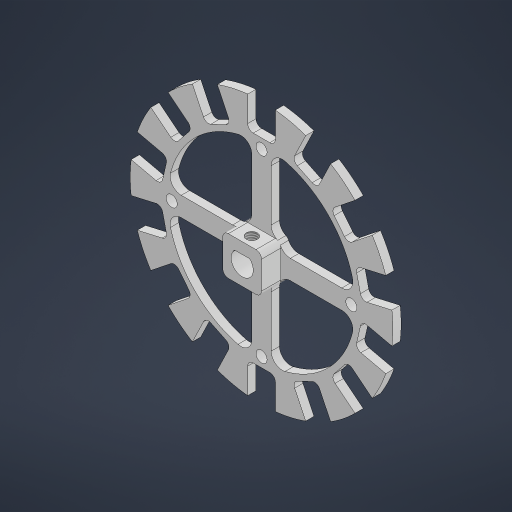
# Autodesk Inventor part: OmniFrame_A
Saved by Autodesk Inventor 2024.2 (Build 282272000, 272)
## iProperties
Created: 2023-12-20
Part Number: OmniFrame_A
Material: 一般
Document SubType Name: Modeling
Designer: Hanaoka
Density: 1 g/cm^3
Appearance: 既定
Author: Hanaoka
Autodesk Inventor part; units mm, degrees
ref_plane "YZ Plane" through (0, 0, 0) normal (1, 0, 0) x (0, 1, 0)
ref_plane "XZ Plane" through (0, 0, 0) normal (0, 1, 0) x (-1, 0, 0)
ref_plane "XY Plane" through (0, 0, 0) normal (0, 0, 1) x (1, 0, 0)
derived "OmniFrame_B.ipt"
sketch "スケッチ1" plane through (0, 0, 0) normal (0, 0, 1) x (1, 0, 0)
  circle A0 centre (0, 0) radius 25 construction
  line L0 (-2.5, 24.874686) -> (-2.5, 19)
  line L1 (-1.5, 18) -> (1.5, 18)
  line L2 (2.5, 19) -> (2.5, 24.874686)
  line L3 (0, 25) -> (0, 18) construction
  line L4 (-2.5, 23.025) -> (-3, 23.025)
  line L5 (-4, 22.025) -> (-4, 21.975)
  line L6 (-3, 20.975) -> (-2.5, 20.975)
  line L7 (2.5, 23.025) -> (3, 23.025)
  line L8 (4, 22.025) -> (4, 21.975)
  line L9 (3, 20.975) -> (2.5, 20.975)
  arc A1 (-3, 23.025) -> (-4, 22.025) centre (-3, 22.025) ccw
  arc A2 (-4, 21.975) -> (-3, 20.975) centre (-3, 21.975) ccw
  arc A3 (4, 22.025) -> (3, 23.025) centre (3, 22.025) ccw
  arc A4 (3, 20.975) -> (4, 21.975) centre (3, 21.975) ccw
  arc A5 (-2.5, 19) -> (-1.5, 18) centre (-1.5, 19) ccw
  arc A6 (1.5, 18) -> (2.5, 19) centre (1.5, 19) ccw
  arc A7 (-10.496213, 16.033699) -> (-9.161361, 15.566614) centre (-9.595244, 16.467583) ccw
  arc A8 (-6.458454, 16.868265) -> (-5.991369, 18.203118) centre (-6.892338, 17.769234) ccw
  line L10 (-9.161361, 15.566614) -> (-6.458454, 16.868265)
  line L11 (-6.397805, 20.199473) -> (-6.848289, 19.982531)
  arc A9 (-6.397805, 20.199473) -> (-5.93072, 21.534326) centre (-6.831689, 21.100442) ccw
  line L12 (-5.952414, 21.579374) -> (-5.93072, 21.534326)
  arc A10 (-5.952414, 21.579374) -> (-7.287266, 22.046459) centre (-6.853383, 21.145491) ccw
  line L13 (-7.737751, 21.829518) -> (-7.287266, 22.046459)
  line L14 (-11.803618, 17.596171) -> (-11.353134, 17.813113)
  line L15 (-5.991369, 18.203118) -> (-8.5403, 23.496027)
  line L16 (-10.847093, 22.524222) -> (-7.809907, 16.21744) construction
  line L17 (-13.045144, 21.326608) -> (-10.496213, 16.033699)
  arc A11 (-13.138471, 18.063256) -> (-11.803618, 17.596171) centre (-12.237502, 18.49714) ccw
  line L18 (-12.242595, 19.660099) -> (-12.69308, 19.443157)
  line L19 (-13.160165, 18.108304) -> (-13.138471, 18.063256)
  arc A12 (-12.69308, 19.443157) -> (-13.160165, 18.108304) centre (-12.259196, 18.542188) ccw
  arc A13 (-16.413523, 9.891728) -> (-15.008201, 10.050069) centre (-15.790033, 10.673559) ccw
  arc A14 (-13.137732, 12.395564) -> (-13.296074, 13.800885) centre (-13.919563, 13.019053) ccw
  line L20 (-15.008201, 10.050069) -> (-13.137732, 12.395564)
  line L21 (-14.528446, 15.423193) -> (-14.840191, 15.032277)
  arc A15 (-14.528446, 15.423193) -> (-14.686788, 16.828514) centre (-15.310277, 16.046683) ccw
  line L22 (-14.725879, 16.859689) -> (-14.686788, 16.828514)
  arc A16 (-14.725879, 16.859689) -> (-16.1312, 16.701347) centre (-15.349369, 16.077857) ccw
  line L23 (-16.442945, 16.310431) -> (-16.1312, 16.701347)
  line L24 (-18.269385, 10.732204) -> (-17.95764, 11.12312)
  line L25 (-13.296074, 13.800885) -> (-17.889088, 17.463692)
  line L26 (-19.545787, 15.587245) -> (-14.072967, 11.222816) construction
  line L27 (-21.006537, 13.554534) -> (-16.413523, 9.891728)
  arc A17 (-19.674706, 10.573862) -> (-18.269385, 10.732204) centre (-19.051216, 11.355694) ccw
  line L28 (-19.560394, 12.401274) -> (-19.872139, 12.010358)
  line L29 (-19.713798, 10.605037) -> (-19.674706, 10.573862)
  arc A18 (-19.872139, 12.010358) -> (-19.713798, 10.605037) centre (-19.090308, 11.386868) ccw
  arc A19 (-19.079933, 1.790578) -> (-17.882484, 2.542985) centre (-18.857412, 2.765506) ccw
  arc A20 (-17.214921, 5.467769) -> (-17.967328, 6.665218) centre (-18.189849, 5.69029) ccw
  line L30 (-17.882484, 2.542985) -> (-17.214921, 5.467769)
  line L31 (-19.78155, 7.59216) -> (-19.892811, 7.104696)
  arc A21 (-19.78155, 7.59216) -> (-20.533957, 8.789609) centre (-20.756478, 7.814681) ccw
  line L32 (-20.582704, 8.800735) -> (-20.533957, 8.789609)
  arc A22 (-20.582704, 8.800735) -> (-21.780152, 8.048328) centre (-20.805224, 7.825807) ccw
  line L33 (-21.891413, 7.560864) -> (-21.780152, 8.048328)
  line L34 (-21.116676, 1.742593) -> (-21.005415, 2.230057)
  line L35 (-17.967328, 6.665218) -> (-23.694723, 7.972458)
  line L36 (-24.373198, 5.563023) -> (-17.548702, 4.005377) construction
  line L37 (-24.807328, 3.097819) -> (-19.079933, 1.790578)
  arc A23 (-22.314125, 0.990186) -> (-21.116676, 1.742593) centre (-22.091604, 1.965114) ccw
  line L38 (-23.004018, 2.686225) -> (-23.115278, 2.198761)
  line L39 (-22.362871, 1.001312) -> (-22.314125, 0.990186)
  arc A24 (-23.115278, 2.198761) -> (-22.362871, 1.001312) centre (-22.14035, 1.97624) ccw
  arc A25 (-17.967328, -6.665218) -> (-17.214921, -5.467769) centre (-18.189849, -5.69029) ccw
  arc A26 (-17.882484, -2.542985) -> (-19.079933, -1.790578) centre (-18.857412, -2.765506) ccw
  line L40 (-17.214921, -5.467769) -> (-17.882484, -2.542985)
  line L41 (-21.116676, -1.742593) -> (-21.005415, -2.230057)
  arc A27 (-21.116676, -1.742593) -> (-22.314125, -0.990186) centre (-22.091604, -1.965114) ccw
  line L42 (-22.362871, -1.001312) -> (-22.314125, -0.990186)
  arc A28 (-22.362871, -1.001312) -> (-23.115278, -2.198761) centre (-22.14035, -1.97624) ccw
  line L43 (-23.004018, -2.686225) -> (-23.115278, -2.198761)
  line L44 (-19.78155, -7.59216) -> (-19.892811, -7.104696)
  line L45 (-19.079933, -1.790578) -> (-24.807328, -3.097819)
  line L46 (-24.373198, -5.563023) -> (-17.548702, -4.005377) construction
  line L47 (-23.694723, -7.972458) -> (-17.967328, -6.665218)
  arc A29 (-20.533957, -8.789609) -> (-19.78155, -7.59216) centre (-20.756478, -7.814681) ccw
  line L48 (-21.891413, -7.560864) -> (-21.780152, -8.048328)
  line L49 (-20.582704, -8.800735) -> (-20.533957, -8.789609)
  arc A30 (-21.780152, -8.048328) -> (-20.582704, -8.800735) centre (-20.805224, -7.825807) ccw
  arc A31 (-13.296074, -13.800885) -> (-13.137732, -12.395564) centre (-13.919563, -13.019053) ccw
  arc A32 (-15.008201, -10.050069) -> (-16.413523, -9.891728) centre (-15.790033, -10.673559) ccw
  line L50 (-13.137732, -12.395564) -> (-15.008201, -10.050069)
  line L51 (-18.269385, -10.732204) -> (-17.95764, -11.12312)
  arc A33 (-18.269385, -10.732204) -> (-19.674706, -10.573862) centre (-19.051216, -11.355694) ccw
  line L52 (-19.713798, -10.605037) -> (-19.674706, -10.573862)
  arc A34 (-19.713798, -10.605037) -> (-19.872139, -12.010358) centre (-19.090308, -11.386868) ccw
  line L53 (-19.560394, -12.401274) -> (-19.872139, -12.010358)
  line L54 (-14.528446, -15.423193) -> (-14.840191, -15.032277)
  line L55 (-16.413523, -9.891728) -> (-21.006537, -13.554534)
  line L56 (-19.545787, -15.587245) -> (-14.072967, -11.222816) construction
  line L57 (-17.889088, -17.463692) -> (-13.296074, -13.800885)
  arc A35 (-14.686788, -16.828514) -> (-14.528446, -15.423193) centre (-15.310277, -16.046683) ccw
  line L58 (-16.442945, -16.310431) -> (-16.1312, -16.701347)
  line L59 (-14.725879, -16.859689) -> (-14.686788, -16.828514)
  arc A36 (-16.1312, -16.701347) -> (-14.725879, -16.859689) centre (-15.349369, -16.077857) ccw
  arc A37 (-5.991369, -18.203118) -> (-6.458454, -16.868265) centre (-6.892338, -17.769234) ccw
  arc A38 (-9.161361, -15.566614) -> (-10.496213, -16.033699) centre (-9.595244, -16.467583) ccw
  line L60 (-6.458454, -16.868265) -> (-9.161361, -15.566614)
  line L61 (-11.803618, -17.596171) -> (-11.353134, -17.813113)
  arc A39 (-11.803618, -17.596171) -> (-13.138471, -18.063256) centre (-12.237502, -18.49714) ccw
  line L62 (-13.160165, -18.108304) -> (-13.138471, -18.063256)
  arc A40 (-13.160165, -18.108304) -> (-12.69308, -19.443157) centre (-12.259196, -18.542188) ccw
  line L63 (-12.242595, -19.660099) -> (-12.69308, -19.443157)
  line L64 (-6.397805, -20.199473) -> (-6.848289, -19.982531)
  line L65 (-10.496213, -16.033699) -> (-13.045144, -21.326608)
  line L66 (-10.847093, -22.524222) -> (-7.809907, -16.21744) construction
  line L67 (-8.5403, -23.496027) -> (-5.991369, -18.203118)
  arc A41 (-5.93072, -21.534326) -> (-6.397805, -20.199473) centre (-6.831689, -21.100442) ccw
  line L68 (-7.737751, -21.829518) -> (-7.287266, -22.046459)
  line L69 (-5.952414, -21.579374) -> (-5.93072, -21.534326)
  arc A42 (-7.287266, -22.046459) -> (-5.952414, -21.579374) centre (-6.853383, -21.145491) ccw
  arc A43 (2.5, -19) -> (1.5, -18) centre (1.5, -19) ccw
  arc A44 (-1.5, -18) -> (-2.5, -19) centre (-1.5, -19) ccw
  line L70 (1.5, -18) -> (-1.5, -18)
  line L71 (-3, -20.975) -> (-2.5, -20.975)
  arc A45 (-3, -20.975) -> (-4, -21.975) centre (-3, -21.975) ccw
  line L72 (-4, -22.025) -> (-4, -21.975)
  arc A46 (-4, -22.025) -> (-3, -23.025) centre (-3, -22.025) ccw
  line L73 (-2.5, -23.025) -> (-3, -23.025)
  line L74 (3, -20.975) -> (2.5, -20.975)
  line L75 (-2.5, -19) -> (-2.5, -24.874686)
  line L76 (0, -25) -> (0, -18) construction
  line L77 (2.5, -24.874686) -> (2.5, -19)
  arc A47 (4, -21.975) -> (3, -20.975) centre (3, -21.975) ccw
  line L78 (2.5, -23.025) -> (3, -23.025)
  line L79 (4, -22.025) -> (4, -21.975)
  arc A48 (3, -23.025) -> (4, -22.025) centre (3, -22.025) ccw
  arc A49 (10.496213, -16.033699) -> (9.161361, -15.566614) centre (9.595244, -16.467583) ccw
  arc A50 (6.458454, -16.868265) -> (5.991369, -18.203118) centre (6.892338, -17.769234) ccw
  line L80 (9.161361, -15.566614) -> (6.458454, -16.868265)
  line L81 (6.397805, -20.199473) -> (6.848289, -19.982531)
  arc A51 (6.397805, -20.199473) -> (5.93072, -21.534326) centre (6.831689, -21.100442) ccw
  line L82 (5.952414, -21.579374) -> (5.93072, -21.534326)
  arc A52 (5.952414, -21.579374) -> (7.287266, -22.046459) centre (6.853383, -21.145491) ccw
  line L83 (7.737751, -21.829518) -> (7.287266, -22.046459)
  line L84 (11.803618, -17.596171) -> (11.353134, -17.813113)
  line L85 (5.991369, -18.203118) -> (8.5403, -23.496027)
  line L86 (10.847093, -22.524222) -> (7.809907, -16.21744) construction
  line L87 (13.045144, -21.326608) -> (10.496213, -16.033699)
  arc A53 (13.138471, -18.063256) -> (11.803618, -17.596171) centre (12.237502, -18.49714) ccw
  line L88 (12.242595, -19.660099) -> (12.69308, -19.443157)
  line L89 (13.160165, -18.108304) -> (13.138471, -18.063256)
  arc A54 (12.69308, -19.443157) -> (13.160165, -18.108304) centre (12.259196, -18.542188) ccw
  arc A55 (16.413523, -9.891728) -> (15.008201, -10.050069) centre (15.790033, -10.673559) ccw
  arc A56 (13.137732, -12.395564) -> (13.296074, -13.800885) centre (13.919563, -13.019053) ccw
  line L90 (15.008201, -10.050069) -> (13.137732, -12.395564)
  line L91 (14.528446, -15.423193) -> (14.840191, -15.032277)
  arc A57 (14.528446, -15.423193) -> (14.686788, -16.828514) centre (15.310277, -16.046683) ccw
  line L92 (14.725879, -16.859689) -> (14.686788, -16.828514)
  arc A58 (14.725879, -16.859689) -> (16.1312, -16.701347) centre (15.349369, -16.077857) ccw
  line L93 (16.442945, -16.310431) -> (16.1312, -16.701347)
  line L94 (18.269385, -10.732204) -> (17.95764, -11.12312)
  line L95 (13.296074, -13.800885) -> (17.889088, -17.463692)
  line L96 (19.545787, -15.587245) -> (14.072967, -11.222816) construction
  line L97 (21.006537, -13.554534) -> (16.413523, -9.891728)
  arc A59 (19.674706, -10.573862) -> (18.269385, -10.732204) centre (19.051216, -11.355694) ccw
  line L98 (19.560394, -12.401274) -> (19.872139, -12.010358)
  line L99 (19.713798, -10.605037) -> (19.674706, -10.573862)
  arc A60 (19.872139, -12.010358) -> (19.713798, -10.605037) centre (19.090308, -11.386868) ccw
  arc A61 (19.079933, -1.790578) -> (17.882484, -2.542985) centre (18.857412, -2.765506) ccw
  arc A62 (17.214921, -5.467769) -> (17.967328, -6.665218) centre (18.189849, -5.69029) ccw
  line L100 (17.882484, -2.542985) -> (17.214921, -5.467769)
  line L101 (19.78155, -7.59216) -> (19.892811, -7.104696)
  arc A63 (19.78155, -7.59216) -> (20.533957, -8.789609) centre (20.756478, -7.814681) ccw
  line L102 (20.582704, -8.800735) -> (20.533957, -8.789609)
  arc A64 (20.582704, -8.800735) -> (21.780152, -8.048328) centre (20.805224, -7.825807) ccw
  line L103 (21.891413, -7.560864) -> (21.780152, -8.048328)
  line L104 (21.116676, -1.742593) -> (21.005415, -2.230057)
  line L105 (17.967328, -6.665218) -> (23.694723, -7.972458)
  line L106 (24.373198, -5.563023) -> (17.548702, -4.005377) construction
  line L107 (24.807328, -3.097819) -> (19.079933, -1.790578)
  arc A65 (22.314125, -0.990186) -> (21.116676, -1.742593) centre (22.091604, -1.965114) ccw
  line L108 (23.004018, -2.686225) -> (23.115278, -2.198761)
  line L109 (22.362871, -1.001312) -> (22.314125, -0.990186)
  arc A66 (23.115278, -2.198761) -> (22.362871, -1.001312) centre (22.14035, -1.97624) ccw
  arc A67 (17.967328, 6.665218) -> (17.214921, 5.467769) centre (18.189849, 5.69029) ccw
  arc A68 (17.882484, 2.542985) -> (19.079933, 1.790578) centre (18.857412, 2.765506) ccw
  line L110 (17.214921, 5.467769) -> (17.882484, 2.542985)
  line L111 (21.116676, 1.742593) -> (21.005415, 2.230057)
  arc A69 (21.116676, 1.742593) -> (22.314125, 0.990186) centre (22.091604, 1.965114) ccw
  line L112 (22.362871, 1.001312) -> (22.314125, 0.990186)
  arc A70 (22.362871, 1.001312) -> (23.115278, 2.198761) centre (22.14035, 1.97624) ccw
  line L113 (23.004018, 2.686225) -> (23.115278, 2.198761)
  line L114 (19.78155, 7.59216) -> (19.892811, 7.104696)
  line L115 (19.079933, 1.790578) -> (24.807328, 3.097819)
  line L116 (24.373198, 5.563023) -> (17.548702, 4.005377) construction
  line L117 (23.694723, 7.972458) -> (17.967328, 6.665218)
  arc A71 (20.533957, 8.789609) -> (19.78155, 7.59216) centre (20.756478, 7.814681) ccw
  line L118 (21.891413, 7.560864) -> (21.780152, 8.048328)
  line L119 (20.582704, 8.800735) -> (20.533957, 8.789609)
  arc A72 (21.780152, 8.048328) -> (20.582704, 8.800735) centre (20.805224, 7.825807) ccw
  arc A73 (13.296074, 13.800885) -> (13.137732, 12.395564) centre (13.919563, 13.019053) ccw
  arc A74 (15.008201, 10.050069) -> (16.413523, 9.891728) centre (15.790033, 10.673559) ccw
  line L120 (13.137732, 12.395564) -> (15.008201, 10.050069)
  line L121 (18.269385, 10.732204) -> (17.95764, 11.12312)
  arc A75 (18.269385, 10.732204) -> (19.674706, 10.573862) centre (19.051216, 11.355694) ccw
  line L122 (19.713798, 10.605037) -> (19.674706, 10.573862)
  arc A76 (19.713798, 10.605037) -> (19.872139, 12.010358) centre (19.090308, 11.386868) ccw
  line L123 (19.560394, 12.401274) -> (19.872139, 12.010358)
  line L124 (14.528446, 15.423193) -> (14.840191, 15.032277)
  line L125 (16.413523, 9.891728) -> (21.006537, 13.554534)
  line L126 (19.545787, 15.587245) -> (14.072967, 11.222816) construction
  line L127 (17.889088, 17.463692) -> (13.296074, 13.800885)
  arc A77 (14.686788, 16.828514) -> (14.528446, 15.423193) centre (15.310277, 16.046683) ccw
  line L128 (16.442945, 16.310431) -> (16.1312, 16.701347)
  line L129 (14.725879, 16.859689) -> (14.686788, 16.828514)
  arc A78 (16.1312, 16.701347) -> (14.725879, 16.859689) centre (15.349369, 16.077857) ccw
  arc A79 (5.991369, 18.203118) -> (6.458454, 16.868265) centre (6.892338, 17.769234) ccw
  arc A80 (9.161361, 15.566614) -> (10.496213, 16.033699) centre (9.595244, 16.467583) ccw
  line L130 (6.458454, 16.868265) -> (9.161361, 15.566614)
  line L131 (11.803618, 17.596171) -> (11.353134, 17.813113)
  arc A81 (11.803618, 17.596171) -> (13.138471, 18.063256) centre (12.237502, 18.49714) ccw
  line L132 (13.160165, 18.108304) -> (13.138471, 18.063256)
  arc A82 (13.160165, 18.108304) -> (12.69308, 19.443157) centre (12.259196, 18.542188) ccw
  line L133 (12.242595, 19.660099) -> (12.69308, 19.443157)
  line L134 (6.397805, 20.199473) -> (6.848289, 19.982531)
  line L135 (10.496213, 16.033699) -> (13.045144, 21.326608)
  line L136 (10.847093, 22.524222) -> (7.809907, 16.21744) construction
  line L137 (8.5403, 23.496027) -> (5.991369, 18.203118)
  arc A83 (5.93072, 21.534326) -> (6.397805, 20.199473) centre (6.831689, 21.100442) ccw
  line L138 (7.737751, 21.829518) -> (7.287266, 22.046459)
  line L139 (5.952414, 21.579374) -> (5.93072, 21.534326)
  arc A84 (7.287266, 22.046459) -> (5.952414, 21.579374) centre (6.853383, 21.145491) ccw
  circle A85 centre (0, 0) radius 23.75
  circle A86 centre (0, 0) radius 17
  circle A87 centre (0, 0) radius 2
  line L140 (-2.5, -3.5) -> (2.5, -3.5)
  line L141 (3.5, -2.5) -> (3.5, 2.5)
  line L142 (2.5, 3.5) -> (-2.5, 3.5)
  line L143 (-3.5, 2.5) -> (-3.5, -2.5)
  line L144 (-3.5, -3.5) -> (3.5, 3.5) construction
  line L145 (3.5, -3.5) -> (-3.5, 3.5) construction
  arc A88 (-2.5, 3.5) -> (-3.5, 2.5) centre (-2.5, 2.5) ccw
  arc A89 (-3.5, -2.5) -> (-2.5, -3.5) centre (-2.5, -2.5) ccw
  arc A90 (2.5, -3.5) -> (3.5, -2.5) centre (2.5, -2.5) ccw
  arc A91 (3.5, 2.5) -> (2.5, 3.5) centre (2.5, 2.5) ccw
  line L146 (-1.75, 16.909687) -> (-1.75, 3.5)
  line L147 (1.75, 3.5) -> (1.75, 16.909687)
  circle A92 centre (0, 16.25) radius 1
  line L148 (0, -35) -> (0, 35)
  circle A93 centre (0, 16.25) radius 1.75
  circle A94 centre (-16.25, 0) radius 1
  line L149 (-3.5, 1.75) -> (-16.909687, 1.75)
  line L150 (-16.909687, -1.75) -> (-3.5, -1.75)
  circle A95 centre (0, -16.25) radius 1
  line L151 (-1.75, -3.5) -> (-1.75, -16.909687)
  line L152 (1.75, -16.909687) -> (1.75, -3.5)
  circle A96 centre (16.25, 0) radius 1
  line L153 (3.5, -1.75) -> (16.909687, -1.75)
  line L154 (16.909687, 1.75) -> (3.5, 1.75)
  circle A97 centre (-16.25, 0) radius 1.75
  circle A98 centre (0, -16.25) radius 1.75
  circle A99 centre (16.25, 0) radius 1.75
  line L155 (-1.322876, 1.5) -> (1.322876, 1.5)
  point P0 (-2.5, 18)
  point P1 (2.5, 18)
  point P2 (4, 23.025)
  point P3 (4, 20.975)
  point P4 (-4, 22)
  point P5 (-10.062329, 15.13273)
  point P6 (-5.557485, 17.302149)
  point P7 (-5.496836, 20.633357)
  point P8 (-6.386298, 22.480343)
  point P9 (-13.149318, 18.08578)
  point P10 (-15.631691, 9.268238)
  point P11 (-12.514242, 13.177395)
  point P12 (-13.904956, 16.205025)
  point P13 (-15.507711, 17.483179)
  point P14 (-19.694252, 10.58945)
  point P15 (-18.105005, 1.568057)
  point P16 (-16.9924, 6.442697)
  point P17 (-19.559029, 8.567088)
  point P18 (-21.557631, 9.023256)
  point P19 (-22.338498, 0.995749)
  point P20 (-16.9924, -6.442697)
  point P21 (-18.105005, -1.568057)
  point P22 (-21.339197, -0.767665)
  point P23 (-23.337799, -1.223833)
  point P24 (-20.55833, -8.795172)
  point P25 (-12.514242, -13.177395)
  point P26 (-15.631691, -9.268238)
  point P27 (-18.892875, -9.950373)
  point P28 (-20.495629, -11.228527)
  point P29 (-14.706333, -16.844102)
  point P30 (-5.557485, -17.302149)
  point P31 (-10.062329, -15.13273)
  point P32 (-12.704587, -17.162287)
  point P33 (-13.594049, -19.009273)
  point P34 (-5.941567, -21.55685)
  point P35 (2.5, -18)
  point P36 (-2.5, -18)
  point P37 (-4, -20.975)
  point P38 (-4, -23.025)
  point P39 (4, -22)
  point P40 (10.062329, -15.13273)
  point P41 (5.557485, -17.302149)
  point P42 (5.496836, -20.633357)
  point P43 (6.386298, -22.480343)
  point P44 (13.149318, -18.08578)
  point P45 (15.631691, -9.268238)
  point P46 (12.514242, -13.177395)
  point P47 (13.904956, -16.205025)
  point P48 (15.507711, -17.483179)
  point P49 (19.694252, -10.58945)
  point P50 (18.105005, -1.568057)
  point P51 (16.9924, -6.442697)
  point P52 (19.559029, -8.567088)
  point P53 (21.557631, -9.023256)
  point P54 (22.338498, -0.995749)
  point P55 (16.9924, 6.442697)
  point P56 (18.105005, 1.568057)
  point P57 (21.339197, 0.767665)
  point P58 (23.337799, 1.223833)
  point P59 (20.55833, 8.795172)
  point P60 (12.514242, 13.177395)
  point P61 (15.631691, 9.268238)
  point P62 (18.892875, 9.950373)
  point P63 (20.495629, 11.228527)
  point P64 (14.706333, 16.844102)
  point P65 (5.557485, 17.302149)
  point P66 (10.062329, 15.13273)
  point P67 (12.704587, 17.162287)
  point P68 (13.594049, 19.009273)
  point P69 (5.941567, 21.55685)
  point P70 (-1.615385, -16.923077)
  point P71 (-16.923077, -1.615385)
  point P72 (-16.923077, 1.615385)
  point P73 (-1.615385, 16.923077)
  point P74 (0, 18)
  point P75 (-2.5, 23.618055)
  point P76 (-7.995068, 22.363841)
  point P77 (-12.499912, 20.194423)
  point P78 (-16.906614, 16.680195)
  point P79 (-20.024063, 12.771037)
  point P80 (-22.469598, 7.692831)
  point P81 (-23.582203, 2.818192)
  point P82 (-23.582203, -2.818192)
  point P83 (-22.469598, -7.692831)
  point P84 (-20.024063, -12.771037)
  point P85 (-16.906614, -16.680195)
  point P86 (-12.499912, -20.194423)
  point P87 (-7.995068, -22.363841)
  point P88 (-2.5, -23.618055)
  point P89 (2.5, -23.618055)
  point P90 (7.995068, -22.363841)
  point P91 (12.499912, -20.194423)
  point P92 (16.906614, -16.680195)
  point P93 (20.024063, -12.771037)
  point P94 (22.469598, -7.692831)
  point P95 (23.582203, -2.818192)
  point P96 (23.582203, 2.818192)
  point P97 (22.469598, 7.692831)
  point P98 (20.024063, 12.771037)
  point P99 (16.906614, 16.680195)
  point P100 (12.499912, 20.194423)
  point P101 (7.995068, 22.363841)
  point P102 (2.5, 23.618055)
  point P103 (1.615385, 16.923077)
  point P104 (16.923077, 1.615385)
  point P105 (16.923077, -1.615385)
  point P106 (1.615385, -16.923077)
  point P107 (1.75, -16.25)
  point P108 (1.75, -3.5)
  point P109 (-1.75, -3.5)
  point P110 (-1.75, -16.25)
  point P111 (-16.909687, 1.75)
  point P112 (-16.909687, -1.75)
  point P113 (-3.5, -1.75)
  point P114 (3.5, -1.75)
  point P115 (3.5, 1.75)
extrude "押し出し1" add sketch "スケッチ1" along normal blind 1.5 contours L4 A1 L5 A2 L6 L0 A5 L1 A93 A86 A97 A98 L70 A44 L75 L71 A45 L72 A46 L73 A85 L67 L68 A42 L69 A41 L64 A37 L60 A38 L65 L61 A39 L62 A40 L63 L57 L58 A36 L59 A35 L54 A31 L50 A32 L55 L51 A33 L52 A34 L53 L47 L48 A30 L49 A29 L44 A25 L40 A26 L45 L41 A27 L42 A28 L43 L37 L38 A24 L39 A23 L34 A19 L30 A20 L35 L31 A21 L32 A22 L33 L27 L28 A18 L29 A17 L24 A13 L20 A14 L25 L21 A15 L22 A16 L23 L17 L18 A12 L19 A11 L14 A7 L10 A8 L15 L11 A9 L12 A10 L13 | L0 L6 A2 L5 A1 L4 | A85 L137 L138 A84 L139 A83 L134 A79 L130 A80 L135 L131 A81 L132 A82 L133 L127 L128 A78 L129 A77 L124 A73 L120 A74 L125 L121 A75 L122 A76 L123 L117 L118 A72 L119 A71 L114 A67 L110 A68 L115 L111 A69 L112 A70 L113 L107 L108 A66 L109 A65 L104 A61 L100 A62 L105 L101 A63 L102 A64 L103 L97 L98 A60 L99 A59 L94 A55 L90 A56 L95 L91 A57 L92 A58 L93 L87 L88 A54 L89 A53 L84 A49 L80 A50 L85 L81 A51 L82 A52 L83 L77 L78 A48 L79 A47 L74 A43 L70 A98 A86 A99 A93 L1 A6 L2 L9 A4 L8 A3 L7 | A93 A86 A92 L148 | L148 A92 A86 A93 | L13 A10 L12 A9 L11 L15 | L7 A3 L8 A4 L9 L2 | A93 L148 A92 A86 | A86 L147 A93 | A93 L146 A86 | A86 A92 L148 A93 | L17 L14 A11 L19 A12 L18 | L137 L134 A83 L139 A84 L138 | L147 L142 L148 A93 | A93 L148 L142 L146 | L23 A16 L22 A15 L21 L25 | L133 A82 L132 A81 L131 L135 | A86 A99 L154 | L142 A91 L141 A90 L140 L148 A87 | L149 A97 A86 | L142 L148 A87 L140 A89 L143 A88 | L27 L24 A17 L29 A18 L28 | L127 L124 A77 L129 A78 L128 | A99 A86 A96 | A86 A96 A99 | A99 L153 L141 L154 | A97 A86 A94 | A86 A94 A97 | L149 L143 L150 A97 | L33 A22 L32 A21 L31 L35 | L123 A76 L122 A75 L121 L125 | A99 A86 L153 | L148 L155 A87 | A87 L155 L148 | A97 L150 A86 | L37 L34 A23 L39 A24 L38 | L117 L114 A71 L119 A72 L118 | L43 A28 L42 A27 L41 L45 | L113 A70 L112 A69 L111 L115 | L47 L44 A29 L49 A30 L48 | A98 L148 A95 A86 | A86 A95 L148 A98 | A98 L148 L140 L152 | L148 A98 L151 L140 | A98 L148 A95 A86 | A86 A95 L148 A98 | L53 A34 L52 A33 L51 L55 | L107 L104 A65 L109 A66 L108 | L57 L54 A35 L59 A36 L58 | L103 A64 L102 A63 L101 L105 | L63 A40 L62 A39 L61 L65 | L97 L94 A59 L99 A60 L98 | L67 L64 A41 L69 A42 L68 | L93 A58 L92 A57 L91 L95 | L74 A47 L79 A48 L78 L77 | L75 L73 A46 L72 A45 L71 | L87 L84 A53 L89 A54 L88 | L83 A52 L82 A51 L81 L85 picked at (-0.749889, 1.590768) picked at (0.749889, 1.590768)
extrude "押し出し2" add sketch "スケッチ1" along normal blind 5 contours L142 A91 L141 A90 L140 L148 A87 | L142 L148 A87 L140 A89 L143 A88 | L148 L155 A87 | A87 L155 L148 picked at (-0.749889, 1.590768) picked at (0.749889, 1.590768)
fillet "フィレット1" radius 2 16 edges at (-16.9097, 1.75, 0.75) (-16.9097, -1.75, 0.75) (1.75, 16.9097, 0.75) (-1.75, 16.9097, 0.75) (16.9097, 1.75, 0.75) (16.9097, -1.75, 0.75) (1.6154, -16.9231, 0.75) (-1.6154, -16.9231, 0.75) (1.75, 3.5, 0.75) (3.5, 1.75, 0.75) (3.5, -1.75, 0.75) (1.75, -3.5, 0.75) (-3.5, -1.75, 0.75) (-3.5, 1.75, 0.75) (-1.75, 3.5, 0.75) (-1.75, -3.5, 0.75)
sketch "スケッチ2" plane through (-2.5, 3.5, 1.5) normal (0, 1, 0) x (1, 0, 0)
  circle A0 centre (2.5, -1.75) radius 1
  line L0 (1, 0) -> (0, 0)
  line L1 (0, 0) -> (5, -3.5) construction
  line L2 (0, 0) -> (0, -3.5)
  line L3 (0, -3.5) -> (5.002444, 0) construction
  line L4 (4.25, 0) -> (6.75, 0)
  point P0 (2.5, 1.5)
  point P1 (2.501222, -1.75)
  dimension "d6" = 2
  constraints: 4 end point, 2 coincident, 2 midpoint, 1 centre point, 1 point on line
  measures "d6" diameter of A0
extrude "押し出し3" cut sketch "スケッチ2" against normal up to surface (2 mm away)
thread "ねじ1" size "M2x0.4" class "6H" standard "ANSI Metric M Profile" full length
sketch "スケッチ3" plane through (-2.5, 3.5, 5) normal (0, 0, 1) x (1, 0, 0)
  circle A0 centre (1.339002, -2.47307) radius 0.5
  arc A1 (5, -7) -> (6, -6) centre (5, -6) ccw
  line L0 (6, -6) -> (6, -1)
  arc A2 (6, -1) -> (5, 0) centre (5, -1) ccw
  line L1 (5, 0) -> (0, 0)
  arc A3 (0, 0) -> (-1, -1) centre (0, -1) ccw
  line L2 (-1, -1) -> (-1, -6)
  arc A4 (-1, -6) -> (0, -7) centre (0, -6) ccw
  line L3 (0, -7) -> (5, -7)
  arc A5 (1.177124, -2) -> (3.822876, -2) centre (2.5, -3.5) ccw
  line L4 (1.177124, -2) -> (3.822876, -2)
  circle A6 centre (2.5, -3.5) radius 1.55 construction
  line L5 (2.5, -3.5) -> (2.5, -2) construction
  circle A7 centre (3.660998, -2.47307) radius 0.5
  point P0 (3.822876, -2)
  point P1 (3.822876, -2)
  point P2 (4.150293, -2.370162)
  point P3 (3.499119, -2)
  point P4 (0.849707, -2.370162)
  point P5 (1.500881, -2)
  dimension "d11" = 1
  dimension "d12" = 3.1
  constraints: 2 end point, 1 centre point, 1 coincident, 1 midpoint, 1 symmetric about line, 7 other
extrude "押し出し4" cut sketch "スケッチ3" against normal up to surface (5 mm away) contours L4 A0 | A0 A5 | A7 L4 | A5 A7
